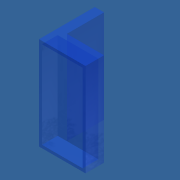
# Autodesk Inventor part: LEGO Brick 4865
Saved by Autodesk Inventor 2011 SP2 (Build 150309200, 309)
## iProperties
Created: 2011-09-27
Part Number: LEGO Brick 4865
Cost Center: 0 kg
Material: Steel
Document SubType Name: Modeling
Designer: BvH
Authority: 0 mm^3
Stock Number: =<Filenr>_<Document number>
Density: 7.85 g/cm^3
Company: Allseas Engineering BV
Subject: =<Title><TITLE 1_2> <TITLE 2_2>
Author: BvH
Act. Code: DW000
SaveDate: 2011-07-28
SaveTime: 18:32
FileName: Standard
TotalMass: 0 kg
TotalVolume: 0 mm^3
Autodesk Inventor part; units mm, degrees
ref_plane "YZ Plane" through (0, 0, 0) normal (1, 0, 0) x (0, 1, 0)
ref_plane "XZ Plane" through (0, 0, 0) normal (0, 1, 0) x (-1, 0, 0)
ref_plane "XY Plane" through (0, 0, 0) normal (0, 0, 1) x (1, 0, 0)
sketch "Sketch1" plane through (0, 0, 0) normal (0, 0, 1) x (1, 0, 0)
  line L0 (-4, 0) -> (4, 0)
  line L1 (4, 0) -> (4, 3.2)
  line L2 (4, 3.2) -> (-2.4, 3.2)
  line L3 (-2.4, 3.2) -> (-2.4, 9.6)
  line L4 (-2.4, 9.6) -> (-4, 9.6)
  line L5 (-4, 9.6) -> (-4, 0)
  point P0 (0, 0)
  point P1 (0, 0)
  dimension "d0" = 8
  dimension "d1" = 3.2
  dimension "d2" = 9.6
  dimension "d3" = 1.6
  constraints: 12 end point, 3 horizontal, 3 vertical, 1 coincident, 1 midpoint
  measures "d0" distance of L0.start L0.end
  measures "d1" distance between parallel lines of L2 L0
  measures "d2" distance between parallel lines of L4 L0
  measures "d3" distance between parallel lines of L5 L3
extrude "Extrusion1" add sketch "Sketch1" along normal mid plane 16
sketch "Sketch2" plane through (-4, 0, 8) normal (0, -1, 0) x (1, 0, 0)
  line L0 (8, 0) -> (0, 0) construction
  line L1 (0, 0) -> (0, -16) construction
  line L2 (0, -16) -> (8, -16) construction
  line L3 (8, -16) -> (8, 0) construction
  line L4 (0.5, -0.5) -> (7.5, -0.5)
  line L5 (7.5, -0.5) -> (7.5, -15.5)
  line L6 (7.5, -15.5) -> (0.5, -15.5)
  line L7 (0.5, -15.5) -> (0.5, -0.5)
  dimension "d6" = 0.5
  constraints: 8 end point, 3 other
  measures "d6" distance between parallel lines of L0 L4
extrude "Extrusion2" cut sketch "Sketch2" against normal blind 2.7
body "Solid1"
